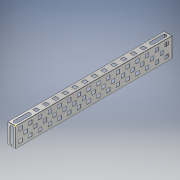
# Autodesk Inventor part: 1sqr x 2sqr metal frame
Saved by Autodesk Inventor 2018 (Build 220112000, 112)
## iProperties
Created: 2018-10-16
Part Number: 1sqr x 2sqr metal frame
Material: Generic
Document SubType Name: Modeling
Designer: USER
Density: 1 g/cm^3
Appearance: Machined - Aluminum
Author: USER
Autodesk Inventor part; units mm, degrees
ref_plane "YZ Plane" through (0, 0, 0) normal (1, 0, 0) x (0, 1, 0)
ref_plane "XZ Plane" through (0, 0, 0) normal (0, 1, 0) x (-1, 0, 0)
ref_plane "XY Plane" through (0, 0, 0) normal (0, 0, 1) x (1, 0, 0)
sketch "Sketch1" plane through (0, 0, 0) normal (1, 0, 0) x (0, 1, 0)
  line L0 (0, 0) -> (-24.9936, 0)
  line L1 (-24.9936, 0) -> (-24.9936, -199.9996)
  line L2 (-24.9936, -199.9996) -> (0, -199.9996)
  line L3 (0, -199.9996) -> (0, 0)
  dimension "d0" = 24.9936
  dimension "d1" = 199.9996
  constraints: 8 end point, 2 parallel, 1 horizontal, 1 perpendicular
  measures "d0" distance of L2.end L1.end
  measures "d1" distance of L1.end L0.end
sketch "Sketch2" plane through (0, 0, 0) normal (0, 1, 0) x (-1, 0, 0)
  line L0 (0, 0) -> (10.0076, 0)
  line L1 (10.0076, 0) -> (10.0076, -199.9996)
  line L2 (10.0076, -199.9996) -> (0, -199.9996)
  line L3 (0, -199.9996) -> (0, 0)
  dimension "d2" = 10.0076
  dimension "d3" = 199.9996
  constraints: 8 end point, 2 parallel, 1 horizontal, 1 perpendicular
  measures "d2" distance of L1.end L2.end
  measures "d3" distance of L0.end L1.end
sketch "Sketch3" plane through (0, 0, 0) normal (0, 0, 1) x (1, 0, 0)
  line L0 (0, 0) -> (-10.0076, 0)
  line L1 (-10.0076, 0) -> (-10.0076, -24.9936)
  line L2 (-10.0076, -24.9936) -> (0, -24.9936)
  line L3 (0, -24.9936) -> (0, 0)
  dimension "d4" = 10.0076
  dimension "d5" = 24.9936
  constraints: 8 end point, 2 parallel, 1 horizontal, 1 perpendicular
  measures "d4" distance of L2.end L1.end
  measures "d5" distance of L1.end L0.end
extrude "Extrusion1" add sketch "Sketch2" against normal blind 0.254
extrude "Extrusion2" add sketch "Sketch1" against normal blind 0.254 separate body
extrude "Extrusion3" add sketch "Sketch3" against normal blind 0.254 separate body
sketch "Sketch4" plane through (0, 0, 0) normal (1, 0, 0) x (0, 0, -1)
  point P0 (0, 0)
sketch "Sketch5" plane through (0, -24.9936, -199.9996) normal (0, 0, -1) x (-1, 0, 0)
  line L0 (0, 0) -> (10.0076, 0)
  line L1 (10.0076, 0) -> (10.0076, 24.9936)
  line L2 (10.0076, 24.9936) -> (0, 24.9936)
  line L3 (0, 24.9936) -> (0, 0)
  dimension "d12" = 10.0076
  dimension "d13" = 24.9936
  constraints: 8 end point, 2 parallel, 1 horizontal, 1 perpendicular
  measures "d12" distance of L2.end L1.end
  measures "d13" distance of L1.end L0.end
extrude "Extrusion4" add sketch "Sketch5" against normal blind 0.254 separate body
sketch "Sketch6" plane through (0, -24.9936, -199.9996) normal (0, 0, -1) x (-1, 0, 0)
  line L0 (4.9724, 20.4485) -> (4.9724, 3.7861) construction
  line L1 (2.5639, 20.4485) -> (2.5639, 3.7861)
  line L2 (7.3809, 3.7861) -> (7.3809, 20.4485)
  arc A0 (7.3809, 20.4485) -> (2.5639, 20.4485) centre (4.9724, 20.4485) ccw
  arc A1 (2.5639, 3.7861) -> (7.3809, 3.7861) centre (4.9724, 3.7861) ccw
  point P0 (0, 24.9936)
  point P1 (4.9724, 12.1173)
  dimension "d16" = 16.6624
  constraints: 8 end point, 4 point on circle, 4 tangent, 2 centre point, 1 midpoint, 1 parallel, 1 vertical
  measures "d16" distance of L0.start L0.end
extrude "Extrusion5" cut sketch "Sketch6" against normal through all bodies 4
sketch "Sketch7" plane through (0, 0, 0) normal (0, 0, 1) x (1, 0, 0)
  arc A0 (-7.3809, -21.2075) -> (-2.5639, -21.2075) centre (-4.9724, -21.2075) ccw projected
  arc A1 (-2.5639, -4.5451) -> (-7.3809, -4.5451) centre (-4.9724, -4.5451) ccw projected
  line L0 (-4.9724, -21.2075) -> (-4.9724, -4.5451) construction
  line L1 (-2.5639, -21.2075) -> (-2.5639, -4.5451)
  line L2 (-7.3809, -4.5451) -> (-7.3809, -21.2075)
  arc A2 (-7.3809, -21.2075) -> (-2.5639, -21.2075) centre (-4.9724, -21.2075) ccw
  arc A3 (-2.5639, -4.5451) -> (-7.3809, -4.5451) centre (-4.9724, -4.5451) ccw
  point P0 (0, 0)
  point P1 (-4.9724, -12.8763)
  dimension "d19" = 16.6624
  constraints: 8 end point, 4 point on circle, 4 tangent, 2 centre point, 1 concentric, 1 midpoint, 1 parallel, 1 vertical
  measures "d19" distance of L0.start L0.end
extrude "Extrusion6" cut sketch "Sketch7" against normal through all bodies 3
sketch "Sketch8" plane through (0, 0, 0) normal (0, 1, 0) x (1, 0, 0)
  line L0 (-4.8736, 4.9634) -> (-4.8736, 21.6258) construction
  line L1 (-2.3489, 4.9634) -> (-2.3489, 21.6258)
  line L2 (-7.3982, 21.6258) -> (-7.3982, 4.9634)
  arc A0 (-7.3982, 4.9634) -> (-2.3489, 4.9634) centre (-4.8736, 4.9634) ccw
  arc A1 (-2.3489, 21.6258) -> (-7.3982, 21.6258) centre (-4.8736, 21.6258) ccw
  line L3 (-10.0076, 0.254) -> (0, 0.254) projected
  line L4 (-5.1165, 178.7958) -> (-5.1165, 195.4582) construction
  line L5 (-2.8347, 178.7958) -> (-2.8347, 195.4582)
  line L6 (-7.3982, 195.4582) -> (-7.3982, 178.7958)
  arc A2 (-7.3982, 178.7958) -> (-2.8347, 178.7958) centre (-5.1165, 178.7958) ccw
  arc A3 (-2.8347, 195.4582) -> (-7.3982, 195.4582) centre (-5.1165, 195.4582) ccw
  line L7 (-10.0076, 0) -> (-10.0076, 199.9996) projected
  line L8 (0, 199.7456) -> (-10.0076, 199.7456) projected
  line L9 (-2.8347, 28.9237) -> (-7.3982, 28.9237)
  line L10 (-7.3982, 28.9237) -> (-7.3982, 33.4972)
  line L11 (-7.3982, 33.4972) -> (-2.8347, 33.4972)
  line L12 (-2.8347, 33.4972) -> (-2.8347, 28.9237)
  line L13 (-7.3982, 41.3697) -> (-7.3982, 45.9432)
  line L14 (-2.8347, 41.3697) -> (-7.3982, 41.3697)
  line L15 (-2.8347, 45.9432) -> (-2.8347, 41.3697)
  line L16 (-7.3982, 45.9432) -> (-2.8347, 45.9432)
  line L17 (-7.3982, 53.8157) -> (-7.3982, 58.3892)
  line L18 (-2.8347, 53.8157) -> (-7.3982, 53.8157)
  line L19 (-2.8347, 58.3892) -> (-2.8347, 53.8157)
  line L20 (-7.3982, 58.3892) -> (-2.8347, 58.3892)
  line L21 (-7.3982, 66.2617) -> (-7.3982, 70.8352)
  line L22 (-2.8347, 66.2617) -> (-7.3982, 66.2617)
  line L23 (-2.8347, 70.8352) -> (-2.8347, 66.2617)
  line L24 (-7.3982, 70.8352) -> (-2.8347, 70.8352)
  line L25 (-7.3982, 78.7077) -> (-7.3982, 83.2812)
  line L26 (-2.8347, 78.7077) -> (-7.3982, 78.7077)
  line L27 (-2.8347, 83.2812) -> (-2.8347, 78.7077)
  line L28 (-7.3982, 83.2812) -> (-2.8347, 83.2812)
  line L29 (-7.3982, 91.1537) -> (-7.3982, 95.7272)
  line L30 (-2.8347, 91.1537) -> (-7.3982, 91.1537)
  line L31 (-2.8347, 95.7272) -> (-2.8347, 91.1537)
  line L32 (-7.3982, 95.7272) -> (-2.8347, 95.7272)
  line L33 (-7.3982, 103.5997) -> (-7.3982, 108.1732)
  line L34 (-2.8347, 103.5997) -> (-7.3982, 103.5997)
  line L35 (-2.8347, 108.1732) -> (-2.8347, 103.5997)
  line L36 (-7.3982, 108.1732) -> (-2.8347, 108.1732)
  line L37 (-7.3982, 116.0457) -> (-7.3982, 120.6192)
  line L38 (-2.8347, 116.0457) -> (-7.3982, 116.0457)
  line L39 (-2.8347, 120.6192) -> (-2.8347, 116.0457)
  line L40 (-7.3982, 120.6192) -> (-2.8347, 120.6192)
  line L41 (-7.3982, 128.4917) -> (-7.3982, 133.0652)
  line L42 (-2.8347, 128.4917) -> (-7.3982, 128.4917)
  line L43 (-2.8347, 133.0652) -> (-2.8347, 128.4917)
  line L44 (-7.3982, 133.0652) -> (-2.8347, 133.0652)
  line L45 (-7.3982, 140.9377) -> (-7.3982, 145.5112)
  line L46 (-2.8347, 140.9377) -> (-7.3982, 140.9377)
  line L47 (-2.8347, 145.5112) -> (-2.8347, 140.9377)
  line L48 (-7.3982, 145.5112) -> (-2.8347, 145.5112)
  line L49 (-7.3982, 153.3837) -> (-7.3982, 157.9572)
  line L50 (-2.8347, 153.3837) -> (-7.3982, 153.3837)
  line L51 (-2.8347, 157.9572) -> (-2.8347, 153.3837)
  line L52 (-7.3982, 157.9572) -> (-2.8347, 157.9572)
  line L53 (-7.3982, 165.8297) -> (-7.3982, 170.4032)
  line L54 (-2.8347, 165.8297) -> (-7.3982, 165.8297)
  line L55 (-2.8347, 170.4032) -> (-2.8347, 165.8297)
  line L56 (-7.3982, 170.4032) -> (-2.8347, 170.4032)
  point P0 (0, 0)
  point P1 (-4.8736, 13.2946)
  point P2 (-5.1165, 187.127)
  dimension "d22" = 16.6624
  dimension "d23" = 2.1848
  dimension "d24" = 16.6624
  dimension "d25" = 2.6094
  dimension "d26" = 2.6094
  dimension "d28" = 4.2874
  dimension "d34" = 12.446
  constraints: 112 end point, 8 point on circle, 8 tangent, 4 centre point, 4 parallel, 3 vertical, 2 midpoint, 1 collinear, 1 horizontal, 1 perpendicular, 87 other
  measures "d22" distance of L0.start L0.end
  measures "d23" distance edge to line of A0 L3
  measures "d24" distance of L4.start L4.end
  measures "d25" distance between parallel lines of L2 L7
  measures "d26" distance between parallel lines of L6 L7
  measures "d28" distance from line of L8 L4.end
  measures "d34" distance of L9.end L13.start
extrude "Extrusion7" cut sketch "Sketch8" against normal through all bodies 1
sketch "Sketch9" plane through (0, 0, 0) normal (1, 0, 0) x (0, 0, -1)
  line L0 (28.9237, -3.3419) -> (33.4957, -3.3419)
  line L1 (33.4957, -3.3419) -> (33.4957, -7.9139)
  line L2 (33.4957, -7.9139) -> (28.9237, -7.9139)
  line L3 (28.9237, -7.9139) -> (28.9237, -3.3419)
  line L4 (41.3697, -7.9139) -> (41.3697, -3.3419)
  line L5 (41.3697, -3.3419) -> (45.9417, -3.3419)
  line L6 (45.9417, -3.3419) -> (45.9417, -7.9139)
  line L7 (45.9417, -7.9139) -> (41.3697, -7.9139)
  line L8 (53.8157, -7.9139) -> (53.8157, -3.3419)
  line L9 (53.8157, -3.3419) -> (58.3877, -3.3419)
  line L10 (58.3877, -3.3419) -> (58.3877, -7.9139)
  line L11 (58.3877, -7.9139) -> (53.8157, -7.9139)
  line L12 (66.2617, -7.9139) -> (66.2617, -3.3419)
  line L13 (66.2617, -3.3419) -> (70.8337, -3.3419)
  line L14 (70.8337, -3.3419) -> (70.8337, -7.9139)
  line L15 (70.8337, -7.9139) -> (66.2617, -7.9139)
  line L16 (78.7077, -7.9139) -> (78.7077, -3.3419)
  line L17 (78.7077, -3.3419) -> (83.2797, -3.3419)
  line L18 (83.2797, -3.3419) -> (83.2797, -7.9139)
  line L19 (83.2797, -7.9139) -> (78.7077, -7.9139)
  line L20 (91.1537, -7.9139) -> (91.1537, -3.3419)
  line L21 (91.1537, -3.3419) -> (95.7257, -3.3419)
  line L22 (95.7257, -3.3419) -> (95.7257, -7.9139)
  line L23 (95.7257, -7.9139) -> (91.1537, -7.9139)
  line L24 (103.5997, -7.9139) -> (103.5997, -3.3419)
  line L25 (103.5997, -3.3419) -> (108.1717, -3.3419)
  line L26 (108.1717, -3.3419) -> (108.1717, -7.9139)
  line L27 (108.1717, -7.9139) -> (103.5997, -7.9139)
  line L28 (116.0457, -7.9139) -> (116.0457, -3.3419)
  line L29 (116.0457, -3.3419) -> (120.6177, -3.3419)
  line L30 (120.6177, -3.3419) -> (120.6177, -7.9139)
  line L31 (120.6177, -7.9139) -> (116.0457, -7.9139)
  line L32 (128.4917, -7.9139) -> (128.4917, -3.3419)
  line L33 (128.4917, -3.3419) -> (133.0637, -3.3419)
  line L34 (133.0637, -3.3419) -> (133.0637, -7.9139)
  line L35 (133.0637, -7.9139) -> (128.4917, -7.9139)
  line L36 (140.9377, -7.9139) -> (140.9377, -3.3419)
  line L37 (140.9377, -3.3419) -> (145.5097, -3.3419)
  line L38 (145.5097, -3.3419) -> (145.5097, -7.9139)
  line L39 (145.5097, -7.9139) -> (140.9377, -7.9139)
  line L40 (153.3837, -7.9139) -> (153.3837, -3.3419)
  line L41 (153.3837, -3.3419) -> (157.9557, -3.3419)
  line L42 (157.9557, -3.3419) -> (157.9557, -7.9139)
  line L43 (157.9557, -7.9139) -> (153.3837, -7.9139)
  line L44 (165.8297, -7.9139) -> (165.8297, -3.3419)
  line L45 (165.8297, -3.3419) -> (170.4017, -3.3419)
  line L46 (170.4017, -3.3419) -> (170.4017, -7.9139)
  line L47 (170.4017, -7.9139) -> (165.8297, -7.9139)
  line L48 (178.2757, -7.9139) -> (178.2757, -3.3419)
  line L49 (178.2757, -3.3419) -> (182.8477, -3.3419)
  line L50 (182.8477, -3.3419) -> (182.8477, -7.9139)
  line L51 (182.8477, -7.9139) -> (178.2757, -7.9139)
  line L52 (190.7217, -7.9139) -> (190.7217, -3.3419)
  line L53 (190.7217, -3.3419) -> (195.2937, -3.3419)
  line L54 (195.2937, -3.3419) -> (195.2937, -7.9139)
  line L55 (195.2937, -7.9139) -> (190.7217, -7.9139)
  line L56 (16.4777, -7.9139) -> (16.4777, -3.3419)
  line L57 (16.4777, -3.3419) -> (21.0497, -3.3419)
  line L58 (21.0497, -3.3419) -> (21.0497, -7.9139)
  line L59 (21.0497, -7.9139) -> (16.4777, -7.9139)
  line L60 (4.0317, -7.9139) -> (4.0317, -3.3419)
  line L61 (4.0317, -3.3419) -> (8.6037, -3.3419)
  line L62 (8.6037, -3.3419) -> (8.6037, -7.9139)
  line L63 (8.6037, -7.9139) -> (4.0317, -7.9139)
  line L64 (0, -24.9936) -> (0, 0) projected
  line L65 (199.9996, 0) -> (199.9996, -24.9936) projected
  line L66 (28.9237, -21.6517) -> (33.4957, -21.6517)
  line L67 (33.4957, -21.6517) -> (33.4957, -17.0797)
  line L68 (33.4957, -17.0797) -> (28.9237, -17.0797)
  line L69 (28.9237, -17.0797) -> (28.9237, -21.6517)
  line L70 (41.3697, -17.0797) -> (41.3697, -21.6517)
  line L71 (41.3697, -21.6517) -> (45.9417, -21.6517)
  line L72 (45.9417, -21.6517) -> (45.9417, -17.0797)
  line L73 (45.9417, -17.0797) -> (41.3697, -17.0797)
  line L74 (53.8157, -17.0797) -> (53.8157, -21.6517)
  line L75 (53.8157, -21.6517) -> (58.3877, -21.6517)
  line L76 (58.3877, -21.6517) -> (58.3877, -17.0797)
  line L77 (58.3877, -17.0797) -> (53.8157, -17.0797)
  line L78 (66.2617, -17.0797) -> (66.2617, -21.6517)
  line L79 (66.2617, -21.6517) -> (70.8337, -21.6517)
  line L80 (70.8337, -21.6517) -> (70.8337, -17.0797)
  line L81 (70.8337, -17.0797) -> (66.2617, -17.0797)
  line L82 (78.7077, -17.0797) -> (78.7077, -21.6517)
  line L83 (78.7077, -21.6517) -> (83.2797, -21.6517)
  line L84 (83.2797, -21.6517) -> (83.2797, -17.0797)
  line L85 (83.2797, -17.0797) -> (78.7077, -17.0797)
  line L86 (91.1537, -17.0797) -> (91.1537, -21.6517)
  line L87 (91.1537, -21.6517) -> (95.7257, -21.6517)
  line L88 (95.7257, -21.6517) -> (95.7257, -17.0797)
  line L89 (95.7257, -17.0797) -> (91.1537, -17.0797)
  line L90 (103.5997, -17.0797) -> (103.5997, -21.6517)
  line L91 (103.5997, -21.6517) -> (108.1717, -21.6517)
  line L92 (108.1717, -21.6517) -> (108.1717, -17.0797)
  line L93 (108.1717, -17.0797) -> (103.5997, -17.0797)
  line L94 (116.0457, -17.0797) -> (116.0457, -21.6517)
  line L95 (116.0457, -21.6517) -> (120.6177, -21.6517)
  line L96 (120.6177, -21.6517) -> (120.6177, -17.0797)
  line L97 (120.6177, -17.0797) -> (116.0457, -17.0797)
  line L98 (128.4917, -17.0797) -> (128.4917, -21.6517)
  line L99 (128.4917, -21.6517) -> (133.0637, -21.6517)
  line L100 (133.0637, -21.6517) -> (133.0637, -17.0797)
  line L101 (133.0637, -17.0797) -> (128.4917, -17.0797)
  line L102 (140.9377, -17.0797) -> (140.9377, -21.6517)
  line L103 (140.9377, -21.6517) -> (145.5097, -21.6517)
  line L104 (145.5097, -21.6517) -> (145.5097, -17.0797)
  line L105 (145.5097, -17.0797) -> (140.9377, -17.0797)
  line L106 (153.3837, -17.0797) -> (153.3837, -21.6517)
  line L107 (153.3837, -21.6517) -> (157.9557, -21.6517)
  line L108 (157.9557, -21.6517) -> (157.9557, -17.0797)
  line L109 (157.9557, -17.0797) -> (153.3837, -17.0797)
  line L110 (165.8297, -17.0797) -> (165.8297, -21.6517)
  line L111 (165.8297, -21.6517) -> (170.4017, -21.6517)
  line L112 (170.4017, -21.6517) -> (170.4017, -17.0797)
  line L113 (170.4017, -17.0797) -> (165.8297, -17.0797)
  line L114 (178.2757, -17.0797) -> (178.2757, -21.6517)
  line L115 (178.2757, -21.6517) -> (182.8477, -21.6517)
  line L116 (182.8477, -21.6517) -> (182.8477, -17.0797)
  line L117 (182.8477, -17.0797) -> (178.2757, -17.0797)
  line L118 (190.7217, -17.0797) -> (190.7217, -21.6517)
  line L119 (190.7217, -21.6517) -> (195.2937, -21.6517)
  line L120 (195.2937, -21.6517) -> (195.2937, -17.0797)
  line L121 (195.2937, -17.0797) -> (190.7217, -17.0797)
  line L122 (16.4777, -17.0797) -> (16.4777, -21.6517)
  line L123 (16.4777, -21.6517) -> (21.0497, -21.6517)
  line L124 (21.0497, -21.6517) -> (21.0497, -17.0797)
  line L125 (21.0497, -17.0797) -> (16.4777, -17.0797)
  line L126 (4.0317, -17.0797) -> (4.0317, -21.6517)
  line L127 (4.0317, -21.6517) -> (8.6037, -21.6517)
  line L128 (8.6037, -21.6517) -> (8.6037, -17.0797)
  line L129 (8.6037, -17.0797) -> (4.0317, -17.0797)
  line L130 (10.3393, -14.6772) -> (10.3393, -10.1052)
  line L131 (10.3393, -10.1052) -> (14.9113, -10.1052)
  line L132 (14.9113, -10.1052) -> (14.9113, -14.6772)
  line L133 (14.9113, -14.6772) -> (10.3393, -14.6772)
  line L134 (22.7853, -10.1052) -> (27.3573, -10.1052)
  line L135 (22.7853, -14.6772) -> (22.7853, -10.1052)
  line L136 (27.3573, -10.1052) -> (27.3573, -14.6772)
  line L137 (27.3573, -14.6772) -> (22.7853, -14.6772)
  line L138 (35.2313, -10.1052) -> (39.8033, -10.1052)
  line L139 (35.2313, -14.6772) -> (35.2313, -10.1052)
  line L140 (39.8033, -10.1052) -> (39.8033, -14.6772)
  line L141 (39.8033, -14.6772) -> (35.2313, -14.6772)
  line L142 (47.6773, -10.1052) -> (52.2493, -10.1052)
  line L143 (47.6773, -14.6772) -> (47.6773, -10.1052)
  line L144 (52.2493, -10.1052) -> (52.2493, -14.6772)
  line L145 (52.2493, -14.6772) -> (47.6773, -14.6772)
  line L146 (60.1233, -10.1052) -> (64.6953, -10.1052)
  line L147 (60.1233, -14.6772) -> (60.1233, -10.1052)
  line L148 (64.6953, -10.1052) -> (64.6953, -14.6772)
  line L149 (64.6953, -14.6772) -> (60.1233, -14.6772)
  line L150 (72.5693, -10.1052) -> (77.1413, -10.1052)
  line L151 (72.5693, -14.6772) -> (72.5693, -10.1052)
  line L152 (77.1413, -10.1052) -> (77.1413, -14.6772)
  line L153 (77.1413, -14.6772) -> (72.5693, -14.6772)
  line L154 (85.0153, -10.1052) -> (89.5873, -10.1052)
  line L155 (85.0153, -14.6772) -> (85.0153, -10.1052)
  line L156 (89.5873, -10.1052) -> (89.5873, -14.6772)
  line L157 (89.5873, -14.6772) -> (85.0153, -14.6772)
  line L158 (97.4613, -10.1052) -> (102.0333, -10.1052)
  line L159 (97.4613, -14.6772) -> (97.4613, -10.1052)
  line L160 (102.0333, -10.1052) -> (102.0333, -14.6772)
  line L161 (102.0333, -14.6772) -> (97.4613, -14.6772)
  line L162 (109.9073, -10.1052) -> (114.4793, -10.1052)
  line L163 (109.9073, -14.6772) -> (109.9073, -10.1052)
  line L164 (114.4793, -10.1052) -> (114.4793, -14.6772)
  line L165 (114.4793, -14.6772) -> (109.9073, -14.6772)
  line L166 (122.3533, -10.1052) -> (126.9253, -10.1052)
  line L167 (122.3533, -14.6772) -> (122.3533, -10.1052)
  line L168 (126.9253, -10.1052) -> (126.9253, -14.6772)
  line L169 (126.9253, -14.6772) -> (122.3533, -14.6772)
  line L170 (134.7993, -10.1052) -> (139.3713, -10.1052)
  line L171 (134.7993, -14.6772) -> (134.7993, -10.1052)
  line L172 (139.3713, -10.1052) -> (139.3713, -14.6772)
  line L173 (139.3713, -14.6772) -> (134.7993, -14.6772)
  line L174 (147.2453, -10.1052) -> (151.8173, -10.1052)
  line L175 (147.2453, -14.6772) -> (147.2453, -10.1052)
  line L176 (151.8173, -10.1052) -> (151.8173, -14.6772)
  line L177 (151.8173, -14.6772) -> (147.2453, -14.6772)
  line L178 (159.6913, -10.1052) -> (164.2633, -10.1052)
  line L179 (159.6913, -14.6772) -> (159.6913, -10.1052)
  line L180 (164.2633, -10.1052) -> (164.2633, -14.6772)
  line L181 (164.2633, -14.6772) -> (159.6913, -14.6772)
  line L182 (172.1373, -10.1052) -> (176.7093, -10.1052)
  line L183 (172.1373, -14.6772) -> (172.1373, -10.1052)
  line L184 (176.7093, -10.1052) -> (176.7093, -14.6772)
  line L185 (176.7093, -14.6772) -> (172.1373, -14.6772)
  line L186 (184.5833, -10.1052) -> (189.1553, -10.1052)
  line L187 (184.5833, -14.6772) -> (184.5833, -10.1052)
  line L188 (189.1553, -10.1052) -> (189.1553, -14.6772)
  line L189 (189.1553, -14.6772) -> (184.5833, -14.6772)
  point P0 (33.4972, 0)
  point P1 (28.9237, 0)
  dimension "d38" = 4.5735
  dimension "d39" = 4.572
  dimension "d40" = 4.572
  dimension "d46" = 12.446
  dimension "d53" = 12.446
  dimension "d60" = 12.446
  constraints: 376 end point, 4 horizontal, 3 collinear, 2 parallel, 1 perpendicular, 229 other
  measures "d38" distance of point (33.497, 0) point (28.924, 0)
  measures "d39" distance of L1.end L2.end
  measures "d40" distance of L0.end L1.end
  measures "d46" distance of L2.end L4.start
  measures "d53" distance of L2.end L56.start
  measures "d60" distance of L131.start L134.start
extrude "Extrusion8" cut sketch "Sketch9" against normal blind 0.254 bodies 2
body "Solid1"
body "Solid2"
body "Solid3"
body "Solid4"
